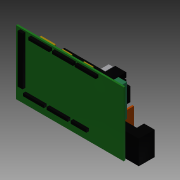
# Autodesk Inventor part: RAMPS1-4
Saved by Autodesk Inventor 2015 (Build 190159000, 159)
## iProperties
Created: 2014-03-14
Part Number: RAMPS1-4
Material: Generic
Document SubType Name: Modeling
Designer: Jack
Density: 1 g/cm^3
Appearance: Default
Author: Jack
Autodesk Inventor part; units mm, degrees
ref_plane "YZ Plane" through (0, 0, 0) normal (1, 0, 0) x (0, 1, 0)
ref_plane "XZ Plane" through (0, 0, 0) normal (0, 1, 0) x (-1, 0, 0)
ref_plane "XY Plane" through (0, 0, 0) normal (0, 0, 1) x (1, 0, 0)
sketch "Sketch1" plane through (0, 0, 0) normal (0, 1, 0) x (-1, 0, 0)
  line L0 (0, 0) -> (101.6, 0)
  line L1 (101.6, 0) -> (101.6, 60.5)
  line L2 (101.6, 60.5) -> (0, 60.5)
  line L3 (0, 60.5) -> (0, 0)
  dimension "d0" = 101.6
  dimension "d1" = 60.5
  constraints: 8 end point, 2 perpendicular, 1 horizontal, 1 parallel
  measures "d0" distance of L0.start L0.end
  measures "d1" distance of L0.end L1.end
extrude "MainBoard" add sketch "Sketch1" along normal blind 1.6
sketch "Sketch2" plane through (0, 1.6, 0) normal (0, 1, 0) x (1, 0, 0)
  line L0 (0, 0) -> (-101.6, 0) projected
  line L1 (-101.6, 0) -> (-101.6, -60.5) projected
  line L2 (0, -60.5) -> (0, 0) projected
  line L3 (-100.6, -1) -> (-100.6, -6)
  line L4 (-100.6, -6) -> (-90, -6)
  line L5 (-90, -6) -> (-90, -1)
  line L6 (-90, -1) -> (-100.6, -1)
  dimension "d4" = 5
  dimension "d5" = 10.6
  dimension "d6" = 1
  dimension "d7" = 1
  constraints: 8 end point, 3 parallel, 1 perpendicular
  measures "d4" distance of L3.start L3.end
  measures "d5" distance of L3.end L4.end
  measures "d6" distance between parallel lines of L0 L6
  measures "d7" distance between parallel lines of L1 L3
extrude "SDPin" add sketch "Sketch2" along normal blind 8.6
sketch "Sketch3" plane through (0, 1.6, 0) normal (0, 1, 0) x (1, 0, 0)
  line L0 (0, -60.5) -> (0, 0) projected
  line L1 (-39.4, -0.1) -> (-39.4, -3.8)
  line L2 (-39.4, -3.8) -> (-31.8, -3.8)
  line L3 (-31.8, -3.8) -> (-31.8, -0.1)
  line L4 (-31.8, -0.1) -> (-39.4, -0.1)
  line L5 (0, 0) -> (-101.6, 0) projected
  dimension "d10" = 3.7
  dimension "d11" = 7.6
  dimension "d12" = 31.8
  dimension "d15" = 0.1
  constraints: 8 end point, 3 parallel, 1 perpendicular
  measures "d10" distance of L1.start L1.end
  measures "d11" distance of L1.end L2.end
  measures "d12" distance between parallel lines of L0 L3
  measures "d15" distance between parallel lines of L5 L4
extrude "ResetSwitch" add sketch "Sketch3" along normal blind 7.6
sketch "Sketch4" plane through (-31.8, 1.6, 0.1) normal (0, 0, -1) x (-1, 0, 0)
  line L0 (7.6, 0) -> (0, 0) projected
  line L1 (0, 0) -> (0, 7.6) projected
  line L2 (2.45, 5) -> (2.45, 2.3)
  line L3 (2.45, 2.3) -> (5.15, 2.3)
  line L4 (5.15, 2.3) -> (5.15, 5)
  line L5 (5.15, 5) -> (2.45, 5)
  point P0 (-31.8, -1.6)
  dimension "d16" = 2.7
  dimension "d17" = 2.7
  dimension "d18" = 2.3
  dimension "d19" = 2.45
  constraints: 8 end point, 2 parallel, 2 perpendicular
  measures "d16" distance of L2.start L2.end
  measures "d17" distance of L2.end L3.end
  measures "d18" distance between parallel lines of L0 L3
  measures "d19" distance between parallel lines of L1 L2
extrude "ResetSwitchProtrusion" add sketch "Sketch4" along normal blind 1.1
sketch "Sketch5" plane through (0, 1.6, 0) normal (0, 1, 0) x (1, 0, 0)
  line L0 (0, 0) -> (-101.6, 0) projected
  line L1 (0, -60.5) -> (0, 0) projected
  line L2 (-19.7, -22.2) -> (-18.2, -22.2)
  line L3 (-18.2, -22.2) -> (-18.2, -5.7)
  line L4 (-18.2, -5.7) -> (-19.7, -5.7)
  line L5 (-19.7, -5.7) -> (-19.7, -22.2)
  dimension "d22" = 1.5
  dimension "d23" = 16.5
  dimension "d24" = 18.2
  dimension "d25" = 5.7
  constraints: 8 end point, 3 perpendicular, 1 parallel
  measures "d22" distance of L2.start L2.end
  measures "d23" distance of L2.end L3.end
  measures "d24" distance between parallel lines of L1 L3
  measures "d25" distance between parallel lines of L0 L4
extrude "FuseLargeFront" add sketch "Sketch5" along normal blind 26.3
sketch "Sketch6" plane through (0, 1.6, 0) normal (0, 1, 0) x (1, 0, 0)
  line L0 (-19.7, -22.2) -> (-19.7, -5.7) projected
  line L1 (0, 0) -> (-101.6, 0) projected
  line L2 (0, -60.5) -> (0, 0) projected
  line L3 (-23.2, -5.7) -> (-23.2, -22.2)
  line L4 (-23.2, -22.2) -> (-21.7, -22.2)
  line L5 (-21.7, -22.2) -> (-21.7, -5.7)
  line L6 (-21.7, -5.7) -> (-23.2, -5.7)
  dimension "d28" = 16.5
  dimension "d29" = 1.5
  dimension "d30" = 2
  dimension "d31" = 5.7
  constraints: 8 end point, 3 perpendicular, 1 parallel
  measures "d28" distance of L3.start L3.end
  measures "d29" distance of L3.end L4.end
  measures "d30" distance between parallel lines of L0 L5
  measures "d31" distance between parallel lines of L1 L6
extrude "FuseSmallBack" add sketch "Sketch6" along normal blind 17.5
sketch "Sketch7" plane through (0, 1.6, 0) normal (0, 1, 0) x (1, 0, 0)
  line L0 (0, 0) -> (-101.6, 0) projected
  line L1 (0, -60.5) -> (0, 0) projected
  line L2 (2.7, -1.5) -> (-9.3, -1.5)
  line L3 (-9.3, -1.5) -> (-9.3, -23.9)
  line L4 (-9.3, -23.9) -> (2.7, -23.9)
  line L5 (2.7, -23.9) -> (2.7, -1.5)
  dimension "d34" = 12
  dimension "d35" = 22.4
  dimension "d36" = 2.7
  dimension "d37" = 1.5
  constraints: 8 end point, 4 perpendicular
  measures "d34" distance of L2.start L2.end
  measures "d35" distance of L2.end L3.end
  measures "d36" distance between parallel lines of L1 L5
  measures "d37" distance between parallel lines of L0 L2
extrude "PowerIn" add sketch "Sketch7" along normal blind 8.1
sketch "Sketch8" plane through (2.7, 1.6, 23.9) normal (1, 0, 0) x (0, 0, -1)
  line L0 (0, 0) -> (22.4, 0) projected
  line L1 (22.4, 0) -> (22.4, 8.1) projected
  line L2 (0, 0) -> (0, 8.1) projected
  line L3 (0, 0) -> (0, 15)
  line L4 (0, 15) -> (22.4, 15)
  line L5 (22.4, 15) -> (22.4, 0)
  point P0 (23.9, -1.6)
  dimension "d40" = 15
  constraints: 6 end point, 1 collinear, 1 perpendicular, 1 point on line
  measures "d40" distance of L0.start L3.end
extrude "PowerInExtension" add sketch "Sketch8" along normal blind 10
sketch "Sketch9" plane through (0, 1.6, 0) normal (0, 1, 0) x (1, 0, 0)
  line L0 (-101.6, -60.5) -> (0, -60.5) projected
  line L1 (0, -60.5) -> (0, -23.9) projected
  line L2 (-100.6, -6) -> (-100.6, -1) projected
  line L3 (-9.1, -54.2) -> (-9.1, -23.9)
  line L4 (-9.1, -23.9) -> (-17.2, -23.9)
  line L5 (-17.2, -23.9) -> (-17.2, -54.2)
  line L6 (-17.2, -54.2) -> (-9.1, -54.2)
  dimension "d43" = 30.3
  dimension "d44" = 8.1
  dimension "d45" = 6.3
  dimension "d46" = 9.1
  constraints: 8 end point, 3 parallel, 1 perpendicular
  measures "d43" distance of L3.start L3.end
  measures "d44" distance of L3.end L4.end
  measures "d45" distance between parallel lines of L0 L6
  measures "d46" distance between parallel lines of L1 L3
extrude "PowerOut" add sketch "Sketch9" along normal blind 10.6
sketch "Sketch10" plane through (0, 1.6, 0) normal (0, 1, 0) x (1, 0, 0)
  line L0 (-101.6, -60.5) -> (0, -60.5) projected
  line L1 (0, -60.5) -> (0, -23.9) projected
  line L2 (0, -23.9) -> (-9.1, -23.9) projected
  line L3 (-27.7, -27.1) -> (-18.1, -27.1)
  line L4 (-18.1, -27.1) -> (-18.1, -40.3)
  line L5 (-18.1, -40.3) -> (-27.7, -40.3)
  line L6 (-27.7, -39.1) -> (-19.3, -39.1)
  line L7 (-19.3, -39.1) -> (-19.3, -28.3)
  line L8 (-19.3, -28.3) -> (-27.7, -28.3)
  line L9 (-27.7, -27.1) -> (-27.7, -28.3)
  line L10 (-27.7, -39.1) -> (-27.7, -40.3)
  dimension "d49" = 9.6
  dimension "d50" = 13.2
  dimension "d51" = 1.2
  dimension "d52" = 20.2
  dimension "d53" = 18.1
  constraints: 16 end point, 4 parallel, 3 perpendicular, 1 collinear, 2 other
  measures "d49" distance of L3.start L3.end
  measures "d50" distance of L3.end L4.end
  measures "d51" distance between parallel lines of L3 L8
  measures "d52" distance between parallel lines of L0 L5
  measures "d53" distance between parallel lines of L1 L4
extrude "MosfetHeatSink" add sketch "Sketch10" along normal blind 22.8
sketch "Sketch11" plane through (0, 1.6, 0) normal (0, 1, 0) x (1, 0, 0)
  line L0 (-101.6, -60.5) -> (0, -60.5) projected
  line L1 (0, -60.5) -> (0, -23.9) projected
  line L2 (0, -23.9) -> (-9.1, -23.9) projected
  line L3 (-19, -52.7) -> (-19, -48.2)
  line L4 (-19, -48.2) -> (-29.3, -48.2)
  line L5 (-29.3, -48.2) -> (-29.3, -52.7)
  line L6 (-29.3, -52.7) -> (-19, -52.7)
  line L7 (-19, -46.7) -> (-19, -42.2)
  line L8 (-19, -42.2) -> (-29.3, -42.2)
  line L9 (-29.3, -42.2) -> (-29.3, -46.7)
  line L10 (-29.3, -46.7) -> (-19, -46.7)
  dimension "d57" = 4.5
  dimension "d58" = 10.3
  dimension "d59" = 4.5
  dimension "d60" = 10.3
  dimension "d61" = 10.5
  dimension "d62" = 7.8
  dimension "d63" = 19
  constraints: 16 end point, 5 perpendicular, 2 parallel, 1 vertical alignment
  measures "d57" distance of L3.start L3.end
  measures "d58" distance of L3.end L4.end
  measures "d59" distance of L10.end L8.start
  measures "d60" distance of L8.start L8.end
  measures "d61" distance between parallel lines of L6 L8
  measures "d62" distance between parallel lines of L0 L6
  measures "d63" distance between parallel lines of L1 L3
extrude "Mosfets" add sketch "Sketch11" along normal blind 19.8
sketch "Sketch12" plane through (0, 0, 0) normal (0, -1, 0) x (1, 0, 0)
  line L0 (-101.6, 60.5) -> (0, 60.5) projected
  line L1 (-101.6, 0) -> (-101.6, 60.5) projected
  line L2 (-97.6, 13.7) -> (-97.6, 59.2)
  line L3 (-97.6, 59.2) -> (-92.8, 59.2)
  line L4 (-92.8, 59.2) -> (-92.8, 13.7)
  line L5 (-92.8, 13.7) -> (-97.6, 13.7)
  dimension "d66" = 45.5
  dimension "d67" = 4.8
  dimension "d68" = 4
  dimension "d69" = 1.3
  constraints: 8 end point, 2 parallel, 2 perpendicular
  measures "d66" distance of L2.start L2.end
  measures "d67" distance of L2.end L3.end
  measures "d68" distance between parallel lines of L1 L2
  measures "d69" distance between parallel lines of L0 L3
extrude "BottomPlugsRear" add sketch "Sketch12" along normal blind 2.6
sketch "Sketch13" plane through (0, 0, 0) normal (0, -1, 0) x (1, 0, 0)
  line L0 (0, 0) -> (-101.6, 0) projected
  line L1 (-101.6, 60.5) -> (0, 60.5) projected
  line L2 (-101.6, 0) -> (-101.6, 60.5) projected
  line L3 (-87.6, 56.6) -> (-87.6, 59)
  line L4 (-87.6, 59) -> (-67.8, 59)
  line L5 (-67.8, 59) -> (-67.8, 56.6)
  line L6 (-67.8, 56.6) -> (-87.6, 56.6)
  line L7 (-65.1, 56.6) -> (-65.1, 59)
  line L8 (-65.1, 59) -> (-45.3, 59)
  line L9 (-45.3, 59) -> (-45.3, 56.6)
  line L10 (-45.3, 56.6) -> (-65.1, 56.6)
  line L11 (-43.6, 56.6) -> (-43.6, 59)
  line L12 (-43.6, 59) -> (-23.8, 59)
  line L13 (-23.8, 59) -> (-23.8, 56.6)
  line L14 (-23.8, 56.6) -> (-43.6, 56.6)
  line L15 (-92.6, 8.3) -> (-92.6, 10.7)
  line L16 (-92.6, 10.7) -> (-72.8, 10.7)
  line L17 (-72.8, 10.7) -> (-72.8, 8.3)
  line L18 (-72.8, 8.3) -> (-92.6, 8.3)
  line L19 (-70.1, 8.3) -> (-70.1, 10.7)
  line L20 (-70.1, 10.7) -> (-50.3, 10.7)
  line L21 (-50.3, 10.7) -> (-50.3, 8.3)
  line L22 (-50.3, 8.3) -> (-70.1, 8.3)
  line L23 (-47.6, 8.3) -> (-47.6, 10.7)
  line L24 (-47.6, 10.7) -> (-32.6, 10.7)
  line L25 (-32.6, 10.7) -> (-32.6, 8.3)
  line L26 (-32.6, 8.3) -> (-47.6, 8.3)
  dimension "d72" = 2.4
  dimension "d73" = 19.8
  dimension "d74" = 2.4
  dimension "d75" = 19.8
  dimension "d76" = 2.4
  dimension "d77" = 19.8
  dimension "d78" = 2.4
  dimension "d79" = 19.8
  dimension "d80" = 2.4
  dimension "d81" = 19.8
  dimension "d82" = 2.4
  dimension "d83" = 15
  dimension "d84" = 1.5
  dimension "d85" = 1.5
  dimension "d86" = 1.5
  dimension "d87" = 8.3
  dimension "d88" = 8.3
  dimension "d89" = 8.3
  dimension "d90" = 14
  dimension "d91" = 2.7
  dimension "d92" = 1.7
  dimension "d93" = 9
  dimension "d94" = 2.7
  dimension "d95" = 2.7
  constraints: 48 end point, 13 parallel, 6 perpendicular
  measures "d72" distance of L3.start L3.end
  measures "d73" distance of L3.end L4.end
  measures "d74" distance of L10.end L8.start
  measures "d75" distance of L8.start L8.end
  measures "d76" distance of L14.end L12.start
  measures "d77" distance of L12.start L12.end
  measures "d78" distance of L18.end L16.start
  measures "d79" distance of L16.start L16.end
  measures "d80" distance of L22.end L20.start
  measures "d81" distance of L20.start L20.end
  measures "d82" distance of L26.end L24.start
  measures "d83" distance of L24.start L24.end
  measures "d84" distance between parallel lines of L1 L12
  measures "d85" distance between parallel lines of L1 L8
  measures "d86" distance between parallel lines of L1 L4
  measures "d87" distance between parallel lines of L0 L18
  measures "d88" distance between parallel lines of L0 L22
  measures "d89" distance between parallel lines of L0 L26
  measures "d90" distance between parallel lines of L2 L3
  measures "d91" distance between parallel lines of L5 L7
  measures "d92" distance between parallel lines of L11 L9
  measures "d93" distance between parallel lines of L2 L15
  measures "d94" distance between parallel lines of L17 L19
  measures "d95" distance between parallel lines of L23 L21
extrude "BottomPlugsSide" add sketch "Sketch13" along normal blind 2.6
sketch "Sketch14" plane through (0, 1.6, 0) normal (0, 1, 0) x (1, 0, 0)
  line L0 (0, 0) -> (-101.6, 0) projected
  line L1 (-101.6, 0) -> (-101.6, -60.5) projected
  line L2 (-101.6, -60.5) -> (0, -60.5) projected
  line L3 (0, -60.5) -> (0, -23.9) projected
  line L4 (0, -23.9) -> (-9.1, -23.9) projected
  line L5 (-37.5, -54) -> (-47.4, -54)
  line L6 (-47.4, -54) -> (-47.4, -51.6)
  line L7 (-47.4, -51.6) -> (-37.5, -51.6)
  line L8 (-37.5, -51.6) -> (-37.5, -54)
  line L9 (-57.6, -54) -> (-67.5, -54)
  line L10 (-67.5, -54) -> (-67.5, -51.6)
  line L11 (-67.5, -51.6) -> (-57.6, -51.6)
  line L12 (-57.6, -51.6) -> (-57.6, -54)
  line L13 (-41.2, -32.2) -> (-51.1, -32.2)
  line L14 (-51.1, -32.2) -> (-51.1, -29.8)
  line L15 (-51.1, -29.8) -> (-41.2, -29.8)
  line L16 (-41.2, -29.8) -> (-41.2, -32.2)
  line L17 (-58.3, -32.2) -> (-68.2, -32.2)
  line L18 (-68.2, -32.2) -> (-68.2, -29.8)
  line L19 (-68.2, -29.8) -> (-58.3, -29.8)
  line L20 (-58.3, -29.8) -> (-58.3, -32.2)
  line L21 (-76.2, -31) -> (-86.1, -31)
  line L22 (-76.2, -28.6) -> (-76.2, -31)
  line L23 (-86.1, -28.6) -> (-76.2, -28.6)
  line L24 (-86.1, -31) -> (-86.1, -28.6)
  line L25 (-76.2, -28.6) -> (-86.1, -28.6)
  line L26 (-76.2, -26.2) -> (-76.2, -28.6)
  line L27 (-86.1, -26.2) -> (-76.2, -26.2)
  line L28 (-86.1, -28.6) -> (-86.1, -26.2)
  line L29 (-76.3, -34.1) -> (-91.3, -34.1)
  line L30 (-91.3, -34.1) -> (-91.3, -36.5)
  line L31 (-91.3, -36.5) -> (-76.3, -36.5)
  line L32 (-76.3, -36.5) -> (-76.3, -34.1)
  line L33 (-73.1, -54.5) -> (-88.1, -54.5)
  line L34 (-88.1, -54.5) -> (-88.1, -47)
  line L35 (-88.1, -47) -> (-73.1, -47)
  line L36 (-73.1, -47) -> (-73.1, -54.5)
  dimension "d98" = 9.9
  dimension "d106" = 6.5
  dimension "d107" = 10.2
  dimension "d108" = 37.5
  dimension "d110" = 33.4
  dimension "d111" = 50.5
  dimension "d116" = 15.5
  dimension "d117" = 31
  dimension "d118" = 2.4
  dimension "d119" = 15
  dimension "d121" = 10.3
  dimension "d122" = 24
  dimension "d123" = 15
  dimension "d124" = 7.5
  dimension "d125" = 6
  dimension "d126" = 13.5
  dimension "d140" = 32.2
  constraints: 64 end point, 15 parallel, 12 perpendicular, 11 equal length, 2 collinear, 2 horizontal alignment
  measures "d98" distance of L5.start L5.end
  measures "d106" distance between parallel lines of L2 L5
  measures "d107" distance between parallel lines of L12 L6
  measures "d108" distance between parallel lines of L8 L3
  measures "d110" distance between parallel lines of L1 L18
  measures "d111" distance between parallel lines of L1 L14
  measures "d116" distance between parallel lines of L1 L24
  measures "d117" distance between parallel lines of L0 L21
  measures "d118" distance of L5.end L6.end
  measures "d119" distance of L29.start L29.end
  measures "d121" distance between parallel lines of L1 L30
  measures "d122" distance between parallel lines of L2 L31
  measures "d123" distance of L33.start L33.end
  measures "d124" distance of L33.end L34.end
  measures "d125" distance between parallel lines of L2 L33
  measures "d126" distance between parallel lines of L1 L34
  measures "d140" distance between parallel lines of L0 L17
extrude "TopPlugs" add sketch "Sketch14" along normal blind 2.6
sketch "Sketch15" plane through (0, 1.6, 0) normal (0, 1, 0) x (1, 0, 0)
  line L0 (0, 0) -> (-101.6, 0) projected
  line L1 (-101.6, 0) -> (-101.6, -60.5) projected
  line L2 (0, -23.9) -> (-9.1, -23.9) projected
  line L3 (-30.2, -25.9) -> (-30.2, -10.9)
  line L4 (-30.2, -10.9) -> (-91.6, -10.9)
  line L5 (-91.6, -10.9) -> (-91.6, -25.9)
  line L6 (-91.6, -25.9) -> (-30.2, -25.9)
  dimension "d129" = 15
  dimension "d130" = 61.4
  dimension "d131" = 10.9
  dimension "d132" = 10
  constraints: 8 end point, 3 perpendicular, 1 parallel
  measures "d129" distance of L3.start L3.end
  measures "d130" distance of L3.end L4.end
  measures "d131" distance between parallel lines of L0 L4
  measures "d132" distance between parallel lines of L1 L5
extrude "StepperDriverBottom" add sketch "Sketch15" along normal blind 14.1
sketch "Sketch16" plane through (0, 1.6, 0) normal (0, 1, 0) x (1, 0, 0)
  line L0 (-76.3, -34.1) -> (-76.3, -36.5) projected
  line L1 (-101.6, 0) -> (-101.6, -60.5) projected
  line L2 (-101.6, -60.5) -> (0, -60.5) projected
  line L3 (0, -23.9) -> (-9.1, -23.9) projected
  line L4 (-29.8, -49.1) -> (-29.8, -34.1)
  line L5 (-29.8, -49.1) -> (-71.6, -49.1)
  line L6 (-71.6, -49.1) -> (-71.6, -34.1)
  line L7 (-71.6, -34.1) -> (-29.8, -34.1)
  dimension "d135" = 15
  dimension "d136" = 41.8
  dimension "d137" = 15
  dimension "d138" = 11.4
  dimension "d139" = 30
  constraints: 8 end point, 2 perpendicular, 1 parallel
  measures "d135" distance of L4.start L4.end
  measures "d136" distance of L4.start L5.end
  measures "d137" distance of L5.end L6.end
  measures "d138" distance between parallel lines of L2 L5
  measures "d139" distance between parallel lines of L1 L6
extrude "StepperDriverTop" add sketch "Sketch16" along normal blind 14.1
sketch "Sketch17" plane through (0, 4.2, 0) normal (0, 1, 0) x (1, 0, 0)
  line L0 (-76.2, -31) -> (-76.2, -26.2) projected
  line L1 (-76.2, -26.2) -> (-86.1, -26.2) projected
  line L2 (-86.1, -26.2) -> (-86.1, -31) projected
  line L3 (-86.1, -31) -> (-76.2, -31) projected
  line L4 (-47.4, -54) -> (-37.5, -54) projected
  line L5 (-37.5, -54) -> (-37.5, -51.6) projected
  line L6 (-37.5, -51.6) -> (-47.4, -51.6) projected
  line L7 (-47.4, -51.6) -> (-47.4, -54) projected
  line L8 (-51.1, -32.2) -> (-41.2, -32.2) projected
  line L9 (-41.2, -32.2) -> (-41.2, -29.8) projected
  line L10 (-41.2, -29.8) -> (-51.1, -29.8) projected
  line L11 (-51.1, -29.8) -> (-51.1, -32.2) projected
  line L12 (-68.2, -32.2) -> (-58.3, -32.2) projected
  line L13 (-58.3, -32.2) -> (-58.3, -29.8) projected
  line L14 (-58.3, -29.8) -> (-68.2, -29.8) projected
  line L15 (-68.2, -29.8) -> (-68.2, -32.2) projected
  line L16 (-67.5, -54) -> (-57.6, -54) projected
  line L17 (-57.6, -54) -> (-57.6, -51.6) projected
  line L18 (-57.6, -51.6) -> (-67.5, -51.6) projected
  line L19 (-67.5, -51.6) -> (-67.5, -54) projected
  line L20 (-88.1, -54.5) -> (-73.1, -54.5) projected
  line L21 (-73.1, -54.5) -> (-73.1, -47) projected
  line L22 (-73.1, -47) -> (-88.1, -47) projected
  line L23 (-88.1, -47) -> (-88.1, -54.5) projected
  line L24 (-76.3, -34.1) -> (-91.3, -34.1) projected
  line L25 (-91.3, -34.1) -> (-91.3, -36.5) projected
  line L26 (-91.3, -36.5) -> (-76.3, -36.5) projected
  line L27 (-76.3, -36.5) -> (-76.3, -34.1) projected
  line L28 (-38, -53.5) -> (-46.9, -53.5)
  line L29 (-46.9, -53.5) -> (-46.9, -52.1)
  line L30 (-46.9, -52.1) -> (-38, -52.1)
  line L31 (-38, -52.1) -> (-38, -53.5)
  line L32 (-58.1, -53.5) -> (-67, -53.5)
  line L33 (-67, -53.5) -> (-67, -52.1)
  line L34 (-67, -52.1) -> (-58.1, -52.1)
  line L35 (-58.1, -52.1) -> (-58.1, -53.5)
  line L36 (-73.6, -54) -> (-87.6, -54)
  line L37 (-87.6, -54) -> (-87.6, -47.5)
  line L38 (-87.6, -47.5) -> (-73.6, -47.5)
  line L39 (-73.6, -47.5) -> (-73.6, -54)
  line L40 (-76.8, -36) -> (-90.8, -36)
  line L41 (-90.8, -36) -> (-90.8, -34.6)
  line L42 (-90.8, -34.6) -> (-76.8, -34.6)
  line L43 (-76.8, -34.6) -> (-76.8, -36)
  line L44 (-76.7, -30.5) -> (-76.7, -26.7)
  line L45 (-76.7, -26.7) -> (-85.6, -26.7)
  line L46 (-85.6, -26.7) -> (-85.6, -30.5)
  line L47 (-85.6, -30.5) -> (-76.7, -30.5)
  line L48 (-58.8, -31.7) -> (-67.7, -31.7)
  line L49 (-67.7, -31.7) -> (-67.7, -30.3)
  line L50 (-67.7, -30.3) -> (-58.8, -30.3)
  line L51 (-58.8, -30.3) -> (-58.8, -31.7)
  line L52 (-41.7, -31.7) -> (-50.6, -31.7)
  line L53 (-50.6, -31.7) -> (-50.6, -30.3)
  line L54 (-50.6, -30.3) -> (-41.7, -30.3)
  line L55 (-41.7, -30.3) -> (-41.7, -31.7)
  point P0 (0, 0)
  dimension "d143" = 0.5
  dimension "d144" = 0.5
  dimension "d145" = 0.5
  dimension "d146" = 0.5
  dimension "d147" = 0.5
  dimension "d148" = 0.5
  dimension "d149" = 0.5
  constraints: 56 end point, 21 other
  measures "d143" distance between parallel lines of L9 L55
  measures "d144" distance between parallel lines of L13 L51
  measures "d145" distance between parallel lines of L27 L43
  measures "d146" distance between parallel lines of L0 L44
  measures "d147" distance between parallel lines of L21 L39
  measures "d148" distance between parallel lines of L17 L35
  measures "d149" distance between parallel lines of L5 L31
extrude "TopPlugConnectors" add sketch "Sketch17" along normal blind 5.5 contours L28 L29 L30 L31 | L32 L33 L34 L35 | L36 L37 L38 L39 | L40 L41 L42 L43 | L47 L46 L45 L44 | L48 L49 L50 L51 | L52 L53 L54 L55
sketch "Sketch18" plane through (0, 15.7, 0) normal (0, 1, 0) x (1, 0, 0)
  line L0 (-30.2, -25.9) -> (-30.2, -10.9) projected
  line L1 (-30.2, -10.9) -> (-91.6, -10.9) projected
  line L2 (-91.6, -10.9) -> (-91.6, -25.9) projected
  line L3 (-91.6, -25.9) -> (-30.2, -25.9) projected
  line L4 (-29.8, -49.1) -> (-29.8, -34.1) projected
  line L5 (-29.8, -34.1) -> (-71.6, -34.1) projected
  line L6 (-71.6, -34.1) -> (-71.6, -49.1) projected
  line L7 (-71.6, -49.1) -> (-29.8, -49.1) projected
  line L8 (-41.8, -38.6) -> (-37.8, -38.6)
  line L9 (-37.8, -38.6) -> (-37.8, -44.6)
  line L10 (-37.8, -44.6) -> (-41.8, -44.6)
  line L11 (-41.8, -44.6) -> (-41.8, -38.6)
  line L12 (-42.2, -15.4) -> (-38.2, -15.4)
  line L13 (-38.2, -15.4) -> (-38.2, -21.4)
  line L14 (-38.2, -21.4) -> (-42.2, -21.4)
  line L15 (-42.2, -21.4) -> (-42.2, -15.4)
  line L16 (-60.2, -15.4) -> (-56.2, -15.4)
  line L17 (-56.2, -15.4) -> (-56.2, -21.4)
  line L18 (-56.2, -21.4) -> (-60.2, -21.4)
  line L19 (-60.2, -21.4) -> (-60.2, -15.4)
  line L20 (-78.2, -15.4) -> (-74.2, -15.4)
  line L21 (-74.2, -15.4) -> (-74.2, -21.4)
  line L22 (-74.2, -21.4) -> (-78.2, -21.4)
  line L23 (-78.2, -21.4) -> (-78.2, -15.4)
  point P0 (0, 0)
  dimension "d154" = 4
  dimension "d155" = 6
  dimension "d156" = 4
  dimension "d157" = 6
  dimension "d158" = 4
  dimension "d159" = 6
  dimension "d160" = 4
  dimension "d161" = 6
  dimension "d162" = 4.5
  dimension "d163" = 4.5
  dimension "d164" = 8
  dimension "d165" = 14
  dimension "d166" = 14
  dimension "d167" = 8
  constraints: 32 end point, 8 parallel, 4 horizontal, 4 perpendicular, 2 horizontal alignment
  measures "d154" distance of L8.start L9.start
  measures "d155" distance of L11.start L8.start
  measures "d156" distance of L12.start L13.start
  measures "d157" distance of L15.start L12.start
  measures "d158" distance of L16.start L17.start
  measures "d159" distance of L19.start L16.start
  measures "d160" distance of L20.start L21.start
  measures "d161" distance of L23.start L20.start
  measures "d162" distance between parallel lines of L5 L8
  measures "d163" distance between parallel lines of L3 L14
  measures "d164" distance between parallel lines of L0 L13
  measures "d165" distance between parallel lines of L15 L17
  measures "d166" distance between parallel lines of L19 L21
  measures "d167" distance between parallel lines of L4 L9
extrude "Extrusion18" add sketch "Sketch18" along normal blind 12 contours L8 L9 L10 L11 | L12 L13 L14 L15 | L16 L17 L18 L19 | L20 L21 L22 L23
body "Solid1"
